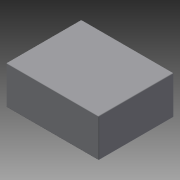
# Autodesk Inventor part: Electrical_Yuasa_Np18-12_Middle
Saved by Autodesk Inventor 2016 SP1 (Build 200210100, 210)
## iProperties
Created: 2010-01-03
Part Number: Electrical_Yuasa_Np18-12_Middle
Document SubType Name: Modeling
Designer: Autodesk
Density: 1 g/cm^3
Material: Generic
Appearance: Default
Mass: 1974.55 g
Surface Area: 1005.79 cm^2
Volume: 1974.55 cm^3
Author: Autodesk
Autodesk Inventor part; units mm, degrees
ref_plane "YZ Plane" through (0, 0, 0) normal (1, 0, 0) x (0, 1, 0)
ref_plane "XZ Plane" through (0, 0, 0) normal (0, 1, 0) x (-1, 0, 0)
ref_plane "XY Plane" through (0, 0, 0) normal (0, 0, 1) x (1, 0, 0)
sketch "Sketch1" plane through (0, 0, 0) normal (0, 0, 1) x (1, 0, 0)
  line L0 (-146.4649, 14.4948) -> (33.1131, 14.4948)
  line L1 (33.1131, 14.4948) -> (33.1131, -60.9432)
  line L2 (33.1131, -60.9432) -> (-146.4649, -60.9432)
  line L3 (-146.4649, -60.9432) -> (-146.4649, 14.4948)
  line L4 (30.5731, 14.7488) -> (-143.9249, 14.7488) projected
  line L5 (-143.9249, -61.1972) -> (30.5731, -61.1972) projected
  line L6 (-147.2269, 11.4468) -> (-147.2269, -57.8952) projected
  point P0 (0, 0)
  point P1 (-146.4649, -23.2242)
  point P2 (-147.2269, -23.2242)
  point P3 (-56.6759, 14.4948)
  point P4 (-56.6759, 14.7488)
  dimension "d0" = 179.578
  dimension "d1" = 75.438
  constraints: 8 end point, 4 midpoint, 2 parallel, 1 horizontal, 1 horizontal alignment, 1 perpendicular, 1 vertical alignment
  measures "d0" distance of L0.start L0.end
  measures "d1" distance of L0.end L1.end
extrude "Extrusion1" add sketch "Sketch1" along normal blind 145.796
fillet "Fillet1" radius 1.27 12 edges at (-146.4649, 14.4948, 72.898) (33.1131, 14.4948, 72.898) (-56.6759, 14.4948, 0) (-56.6759, 14.4948, 145.796) (33.1131, -60.9432, 72.898) (33.1131, -23.2242, 0) (33.1131, -23.2242, 145.796) (-146.4649, -60.9432, 72.898) (-56.6759, -60.9432, 0) (-56.6759, -60.9432, 145.796) (-146.4649, -23.2242, 0) (-146.4649, -23.2242, 145.796)
body "Solid1"
